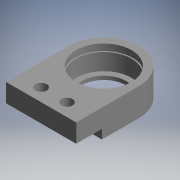
# Autodesk Inventor part: SBGSNA6200ZZ-20_h
Saved by Autodesk Inventor 2017.3 (Build 213256000, 256)
## iProperties
Part Number: SBGSNA6200ZZ-20_h
Material: Generic
Catalog Web Link: www.cadenas.de
Description: BGSNAB, BGSNA, SBGSNA_housing-Bearings with Housings - Front Mount, Shouldered, h selectable/ Retained Bearing
Vendor: MISUMI
Document SubType Name: Modeling
Designer: partserver
Manufacturer: MISUMI
Mass: 14.4753 g
Surface Area: 69.3956 cm^2
Volume: 14.4753 cm^3
Density: 1 g/cm^3
Appearance: PSOLRGB-175-175-175
Category: PARTsolutions
Company: MISUMI
Title: SBGSNA6200ZZ-20
Author: Cadenas PARTsolutions
Comments: Bearings with Housings - Front Mount, Shouldered, h selectable/ Retained Bearing
PSOL_IDENT_0: {$CADENAS_DATA\23d-libs\misumi\metric\12_bearing_holders\bgsna\bgsna_housing.prj},218 {VTYP=3D},{NB=
PSOL_IDENT_1: SBGSNA6200ZZ-20_h},{LINA=SBGSNA6200ZZ-20},{NN=BGSNAB, BGSNA, SBGSNA_housing},{DATE=30.03.2018 01:48:
PSOL_IDENT_2: 32},{GEOMDATE=15.07.2015 02:14:00},{VERSION=},{LINEID=30},{WBVAR=MATB,STH,SEAL,HH,ALT1},{WBNUMERIC=H
PSOL_IDENT_3: H}  {NB=SBGSNA6200ZZ-20_h},{LINA=SBGSNA6200ZZ-20},{KT=DUMMY},{PN=SBGSNA6200ZZ-20},{TYPE=SBGSNA},{MAT
PSOL_IDENT_4: B=SST},{MATBALG= 'ST','Steel','SST','Stainless Steel' },{STH=},{STHALG= '','-' },{ARR=304 Stainless
PSOL_IDENT_5: Steel},{ARRALG=-S},{BN=6200},{SEAL=ZZ},{SEALALG= 'ZZ','ZZ(Double Shielded)','VV','VV(Non-Contact Rub
PSOL_IDENT_6: ber Seal)','DD','DD(Contact Rubber Seal)' },{HH=20},{HHALG=20,25,30},{DD=10},{D=30},{DDHH=24},{B=9},
PSOL_IDENT_7: {H=53.0},{HH1=7},{L=38},{L1=14},{T=15},{T1=10},{DD1=6},{ALT1=},{ALT1ALG= '','Bearing and Retaining R
PSOL_IDENT_8: ing Assembled','NA','with NA (Bearing and Retaining Ring not Assembled)' },{ALT1PN=},{DD2=31.4},{TT=
PSOL_IDENT_9: 1.20},{TIF=1},{M=1.35}
NB: SBGSNA6200ZZ-20_h
NN: BGSNAB, BGSNA, SBGSNA_housing
NT: Bearings with Housings - Front Mount, Shouldered, h selectable/ Retained Bearing
NBSYN: $PN._h
LINA: SBGSNA6200ZZ-20
CATALOG: Misumi
PN: SBGSNA6200ZZ-20
MATB: Stainless Steel
STH: -
ARR: 304 Stainless Steel
BN: 6200
SEAL: ZZ(Double Shielded)
HH: 20
DD: 10
D: 30
DDHH: 24
B: 9
H: 53
HH1: 7
L: 38
L1: 14
T: 15
T1: 10
DD1: 6
ALT1: Bearing and Retaining Ring Assembled
SUPPLIER: MISUMI
ARTICLENO: SBGSNA6200ZZ-20_h
BOMINFO: SBGSNA6200ZZ-20
CREATOR: CADENAS GmbH
Autodesk Inventor part; units mm, degrees
sketch "Sketch_9" plane through (0, 0, 0) normal (0, 0, 1) x (1, 0, 0)
  line L0 (-19, 34) -> (-19, 0)
  line L1 (-19, 0) -> (19, 0)
  line L2 (19, 0) -> (19, 34)
  arc A0 (19, 34) -> (-19, 34) centre (0, 34) ccw
  constraints: 6 end point, 2 point on circle, 1 centre point
extrude "Extrusion1" add sketch "Sketch_9" against normal blind 15
sketch "Sketch_1" plane through (0, 0, 0) normal (1, 0, 0) x (0, 0, -1)
  line L0 (0, 14) -> (0, 0)
  line L1 (0, 0) -> (5, 0)
  line L2 (5, 0) -> (5, 14)
  line L3 (5, 14) -> (0, 14)
  constraints: 8 end point
extrude "Extrusion2" cut sketch "Sketch_1" along normal mid plane 76
sketch "Sketch_2" plane through (0, 0, 0) normal (1, 0, 0) x (0, 0, -1)
  line L0 (15, 34) -> (2, 34)
  line L1 (2, 34) -> (2, 49)
  line L2 (2, 49) -> (11, 49)
  line L3 (11, 49) -> (11, 49.7)
  line L4 (11, 49.7) -> (12.35, 49.7)
  line L5 (12.35, 49.7) -> (12.35, 49)
  line L6 (12.35, 49) -> (15, 49)
  line L7 (15, 49) -> (15, 34)
  line L8 (15, 34) -> (2, 34)
  constraints: 18 end point
revolve "Revolution1" cut sketch "Sketch_2" angle 360 about axis through (0, 34, -15) along (0, 0, -1)
sketch "Sketch4" plane through (0, 0, 0) normal (0, 0, 1) x (1, 0, 0)
  point P0 (0, 34)
hole "Hole1" at (0, 34, 0) direction (0, 0, -1) diameter 24 depth 15
sketch "Sketch5" plane through (0, 0, -15) normal (0, 0, -1) x (-1, 0, 0)
  point P0 (7, 7)
hole "Hole2" at (-7, 7, -15) direction (0, 0, 1) diameter 6 depth 15
pattern_linear "Rectangular Pattern1" count 2 spacing 14 along (1, 0, 0) of "Hole2"
ref_plane "to_bearing_XY" through (0, 34, -6.5) normal (0, 0, -1) x (1, 0, 0)
ref_plane "to_bearing_YZ" through (0, 34, -6.5) normal (1, 0, 0) x (0, -1, 0)
ref_plane "to_bearing_ZX" through (0, 34, -6.5) normal (0, -1, 0) x (0, 0, -1)
ref_plane "to_retaining_ring_XY" through (0, 34, -11) normal (0, 0, 1) x (-1, 0, 0)
ref_plane "to_retaining_ring_YZ" through (0, 34, -11) normal (-1, 0, 0) x (0, -1, 0)
ref_plane "to_retaining_ring_ZX" through (0, 34, -11) normal (0, -1, 0) x (0, 0, 1)
body "Solid1"
